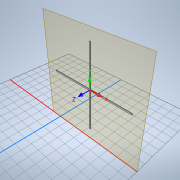
# Autodesk Inventor part: krys
Saved by Autodesk Inventor 2021 (Build 250183000, 183)
## iProperties
Created: 2021-06-22
Part Number: krys
Material: Aluminium
Document SubType Name: Modeling
Designer: Wojciech Wołczek
Mass: 191.849 g
Surface Area: 569.34 cm^2
Volume: 71.055 cm^3
Density: 2.7 g/cm^3
Appearance: Satynowy
Author: Wojciech Wołczek
Autodesk Inventor part; units mm, degrees
ref_plane "YZ Plane" through (0, 0, 0) normal (1, 0, 0) x (0, 1, 0)
ref_plane "XZ Plane" through (0, 0, 0) normal (0, 1, 0) x (-1, 0, 0)
ref_plane "XY Plane" through (0, 0, 0) normal (0, 0, 1) x (1, 0, 0)
ref_plane "Płaszczyzna konstrukcyjna1" through (0, 0, 0) normal (0, 0, 1) x (1, 0, 0)
sketch "Szkic1" plane through (0, 0, 0) normal (0, 0, 1) x (1, 0, 0)
  circle A0 centre (836, 698.5) radius 4 projected
  circle A1 centre (836, 98.5) radius 4 projected
  circle A2 centre (698.5, -39) radius 4 projected
  circle A3 centre (98.5, -39) radius 4 projected
  circle A4 centre (-39, 98.5) radius 4 projected
  circle A5 centre (-39, 698.5) radius 4 projected
  circle A6 centre (836, 398.5) radius 4 projected
  circle A7 centre (398.5, -39) radius 4 projected
  circle A8 centre (-39, 398.5) radius 4 projected
  circle A9 centre (98.5, 836) radius 4 projected
  circle A10 centre (698.5, 836) radius 4 projected
  circle A11 centre (398.5, 836) radius 4 projected
  line L0 (0, 797) -> (0, 0) projected
  line L1 (0, 0) -> (797, 0) projected
  line L2 (797, 0) -> (797, 797) projected
  line L3 (797, 797) -> (0, 797) projected
  line L4 (856, 856) -> (856, -59) projected
  line L5 (856, -59) -> (-59, -59) projected
  line L6 (-59, -59) -> (-59, 856) projected
  line L7 (-59, 856) -> (856, 856) projected
  line L8 (406, 797) -> (391, 797)
  line L9 (391, 797) -> (391, 0)
  line L10 (391, 0) -> (406, 0)
  line L11 (406, 0) -> (406, 797)
  line L12 (406, 797) -> (391, 0) construction
  line L13 (391, 797) -> (406, 0) construction
  line L14 (797, 406) -> (0, 406)
  line L15 (0, 406) -> (0, 391)
  line L16 (0, 391) -> (797, 391)
  line L17 (797, 391) -> (797, 406)
  line L18 (797, 406) -> (0, 391) construction
  line L19 (0, 406) -> (797, 391) construction
  circle A12 centre (761, -24) radius 3 projected
  circle A13 centre (348.5, -24) radius 3 projected
  circle A14 centre (-24, -24) radius 3 projected
  circle A15 centre (-24, 348.5) radius 3 projected
  circle A16 centre (-24, 761) radius 3 projected
  circle A17 centre (248.5, 821) radius 3 projected
  circle A18 centre (648.5, 821) radius 3 projected
  circle A19 centre (821, 648.5) radius 3 projected
  circle A20 centre (821, 248.5) radius 3 projected
  circle A21 centre (821, 348.5) radius 3 projected
  circle A22 centre (821, 761) radius 3 projected
  circle A23 centre (548.5, 821) radius 3 projected
  circle A24 centre (148.5, 821) radius 3 projected
  circle A25 centre (-24, 648.5) radius 3 projected
  circle A26 centre (-24, 248.5) radius 3 projected
  circle A27 centre (36, -24) radius 3 projected
  circle A28 centre (448.5, -24) radius 3 projected
  circle A29 centre (821, -24) radius 3 projected
  circle A30 centre (648.5, -24) radius 3 projected
  circle A31 centre (248.5, -24) radius 3 projected
  circle A32 centre (-24, 36) radius 3 projected
  circle A33 centre (-24, 448.5) radius 3 projected
  circle A34 centre (-24, 821) radius 3 projected
  circle A35 centre (348.5, 821) radius 3 projected
  circle A36 centre (761, 821) radius 3 projected
  circle A37 centre (821, 548.5) radius 3 projected
  circle A38 centre (821, 148.5) radius 3 projected
  circle A39 centre (821, 448.5) radius 3 projected
  circle A40 centre (821, 821) radius 3 projected
  circle A41 centre (448.5, 821) radius 3 projected
  circle A42 centre (36, 821) radius 3 projected
  circle A43 centre (-24, 548.5) radius 3 projected
  circle A44 centre (-24, 148.5) radius 3 projected
  circle A45 centre (148.5, -24) radius 3 projected
  circle A46 centre (548.5, -24) radius 3 projected
  circle A47 centre (821, 36) radius 3 projected
  point P0 (398.5, 398.5)
  point P1 (391, 391)
  point P2 (406, 391)
  point P3 (797, 391)
  point P4 (797, 406)
  point P5 (406, 406)
  point P6 (391, 406)
  point P7 (0, 406)
  dimension "d6" = 15
  dimension "d7" = 797
  dimension "d8" = 15
  constraints: 24 end point, 4 midpoint, 4 parallel, 2 horizontal, 2 perpendicular, 1 point on line
  measures "d6" distance of L10.end L9.end
  measures "d7" distance of L16.end L15.end
  measures "d8" distance of L15.end L14.end
extrude "Wyciągnięcie proste1" add sketch "Szkic1" along normal blind 3 contours L14 L9 L16 L0 | L3 L11 L14 L9 | L14 L11 L16 L9 | L16 L11 L1 L9 | L14 L2 L16 L11
